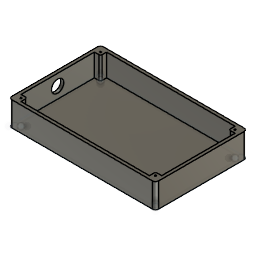
keyboard1_case (Autodesk Fusion 360 design; units mm, degrees)
part number: 2026-01-22-15-28-57-156
part number: 2026-01-22-16-58-12-345
part number: 2026-01-22-17-11-15-376
Autodesk Fusion 360 part; units mm, degrees
note: some values were not read from the file. Set by a fixed rule: which sketch regions a step uses.
sketch "bottom structure" plane through (0, 0, 0) normal (0, 0, 1) x (1, 0, 0)
  line L0 (5, 0) -> (235, 0)
  line L1 (240, 5) -> (240, 145)
  line L2 (235, 150) -> (5, 150)
  line L3 (0, 145) -> (0, 5)
  line L4 (10, 145) -> (230, 145)
  line L5 (235, 140) -> (235, 10)
  line L6 (230, 5) -> (10, 5)
  line L7 (5, 10) -> (5, 140)
  arc A0 (5, 150) -> (0, 145) centre (5, 145) ccw
  arc A1 (10, 145) -> (5, 140) centre (10, 140) ccw
  arc A2 (5, 10) -> (10, 5) centre (10, 10) ccw
  arc A3 (0, 5) -> (5, 0) centre (5, 5) ccw
  arc A4 (235, 140) -> (230, 145) centre (230, 140) ccw
  arc A5 (240, 145) -> (235, 150) centre (235, 145) ccw
  arc A6 (230, 5) -> (235, 10) centre (230, 10) ccw
  arc A7 (235, 0) -> (240, 5) centre (235, 5) ccw
  line L8 (15, 145) -> (15, 137.5)
  line L9 (12.5, 135) -> (5, 135)
  line L10 (225, 145) -> (225, 137.5)
  line L11 (227.5, 135) -> (235, 135)
  line L12 (5, 15) -> (12.5, 15)
  line L13 (15, 12.5) -> (15, 5)
  line L14 (225, 5) -> (225, 12.5)
  line L15 (227.5, 15) -> (235, 15)
  circle A8 centre (230, 10) radius 3
  circle A9 centre (230, 140) radius 3
  circle A10 centre (230, 140) radius 1.35
  circle A11 centre (10, 140) radius 1.35
  circle A12 centre (10, 140) radius 3
  circle A13 centre (230, 10) radius 1.35
  circle A14 centre (10, 10) radius 1.35
  circle A15 centre (10, 10) radius 3
  arc A16 (225, 137.5) -> (227.5, 135) centre (227.5, 137.5) ccw
  arc A17 (227.5, 15) -> (225, 12.5) centre (227.5, 12.5) ccw
  arc A18 (15, 12.5) -> (12.5, 15) centre (12.5, 12.5) ccw
  arc A19 (12.5, 135) -> (15, 137.5) centre (12.5, 137.5) ccw
  point P0 (240, 0)
  point P1 (0, 150)
  point P2 (15, 135)
  point P3 (225, 135)
  point P4 (15, 15)
  point P5 (225, 15)
  dimension "d1" = 150
  dimension "d2" = 240
  dimension "d4" = 5
  dimension "d5" = 5
  dimension "d6" = 5
  dimension "d7" = 5
  dimension "d8" = 5
  dimension "d9" = 5
  dimension "d10" = 5
  dimension "d11" = 5
  dimension "d12" = 5
  dimension "d13" = 5
  dimension "d14" = 5
  dimension "d15" = 5
  dimension "d16" = 10
  dimension "d17" = 10
  dimension "d18" = 10
  dimension "d19" = 10
  dimension "d20" = 10
  dimension "d21" = 10
  dimension "d22" = 10
  dimension "d23" = 10
  dimension "d24" = 5
  dimension "d25" = 6
  dimension "d27" = 5
  dimension "d31" = 6
  dimension "d34" = 2.7
  dimension "d35" = 6
  dimension "d36" = 2.7
  dimension "d38" = 2.7
  dimension "d39" = 6
  dimension "d40" = 2.7
  dimension "d41" = 2.5
  constraint horizontal L0
  constraint vertical L1
  constraint horizontal L2
  constraint vertical L3
  constraint horizontal L4
  constraint vertical L5
  constraint horizontal L6
  constraint vertical L7
  constraint coincident P1 L2
  constraint coincident P1 L3
  constraint tangent L2 A0
  constraint tangent L3 A0
  constraint tangent L4 A1
  constraint tangent L7 A1
  constraint tangent L6 A2
  constraint tangent L7 A2
  constraint coincident origin L0
  constraint coincident origin L3
  constraint tangent L0 A3
  constraint tangent L3 A3
  constraint tangent L4 A4
  constraint tangent L5 A4
  constraint tangent L1 A5
  constraint tangent L2 A5
  constraint tangent L5 A6
  constraint tangent L6 A6
  constraint coincident P0 L0
  constraint coincident P0 L1
  constraint tangent L0 A7
  constraint tangent L1 A7
  constraint coincident L4 L8.start
  constraint perpendicular L4 L8
  constraint coincident L7 L9.end
  constraint perpendicular L7 L9
  constraint coincident L4 L10.start
  constraint perpendicular L4 L10
  constraint coincident L5 L11.end
  constraint perpendicular L5 L11
  constraint coincident L7 L12.start
  constraint perpendicular L7 L12
  constraint coincident L6 L13.end
  constraint perpendicular L6 L13
  constraint coincident L6 L14.start
  constraint perpendicular L6 L14
  constraint coincident L5 L15.end
  constraint perpendicular L5 L15
  constraint coincident P3 L10
  constraint coincident P3 L11
  constraint tangent L10 A16
  constraint tangent L11 A16
  constraint coincident P5 L14
  constraint coincident P5 L15
  constraint tangent L14 A17
  constraint tangent L15 A17
  constraint equal A16 A17
  constraint coincident P4 L12
  constraint coincident P4 L13
  constraint tangent L12 A18
  constraint tangent L13 A18
  constraint equal A16 A18
  constraint coincident P2 L8
  constraint coincident P2 L9
  constraint tangent L8 A19
  constraint tangent L9 A19
  constraint equal A16 A19
  measures "d1" distance of origin P1
  measures "d2" distance of origin P0
  measures "d4" distance of L3 L7
  measures "d5" distance of L1 L5
  measures "d6" distance of L0 L6
  measures "d7" distance of L2 L4
  measures "d8" radius of A0
  measures "d9" radius of A1
  measures "d10" radius of A2
  measures "d11" radius of A3
  measures "d12" radius of A4
  measures "d13" radius of A5
  measures "d14" radius of A6
  measures "d15" radius of A7
  measures "d16" distance of L8.start P2
  measures "d17" distance of P2 L9.end
  measures "d18" distance of L10.start P3
  measures "d19" distance of P3 L11.end
  measures "d20" distance of L12.start P4
  measures "d21" distance of P4 L13.end
  measures "d22" distance of P5 L15.end
  measures "d23" distance of L14.start P5
  measures "d24" horizontal distance of L5.end A6.centre
  measures "d25" diameter of A8
  measures "d27" distance of L6.start A6.centre
  measures "d31" diameter of A9
  measures "d34" diameter of A10
  measures "d35" diameter of A12
  measures "d36" diameter of A11
  measures "d38" diameter of A13
  measures "d39" diameter of A15
  measures "d40" diameter of A14
  measures "d41" radius of A16
extrude "Extrude1" add sketch "bottom structure" along normal blind 40 contours L0 L1 L2 L3 A0 A3 A5 A7 | L4 L7 A1 L8 L9 A19 | L4 L5 A4 L10 L11 A16 | L6 L7 A2 L12 L13 A18 | L5 L6 A6 L14 L15 A17 | A8 | A9 | A12 | A15 makes body 1
sketch "bottom itself" plane through (0, 0, 0) normal (0, 0, 1) x (1, 0, 0)
  line L0 (5, 150) -> (235, 150)
  line L1 (240, 145) -> (240, 5)
  line L2 (235, 0) -> (5, 0)
  line L3 (0, 5) -> (0, 145)
  arc A0 (5, 150) -> (0, 145) centre (5, 145) ccw
  arc A1 (0, 5) -> (5, 0) centre (5, 5) ccw
  arc A2 (235, 0) -> (240, 5) centre (235, 5) ccw
  arc A3 (240, 145) -> (235, 150) centre (235, 145) ccw
  dimension "d44" = 5
  constraint horizontal L0
  constraint vertical L1
  constraint horizontal L2
  constraint vertical L3
  constraint tangent L0 A0
  constraint tangent L3 A0
  constraint tangent L2 A1
  constraint tangent L3 A1
  constraint equal A0 A1
  constraint tangent L1 A2
  constraint tangent L2 A2
  constraint equal A0 A2
  constraint tangent L0 A3
  constraint tangent L1 A3
  constraint equal A0 A3
  measures "d44" radius of A0
extrude "Extrude2" add sketch "bottom itself" along normal blind 5 bodies 1
extrude "Extrude3" cut 1 faces at (84.8596, 54.6296, 5) along direction (0, 0, -1) blind 1.5 on bodies 1 bodies 1
copy_body "Body->Comp1" bodies 1 removing the originals makes body 2 in component "top plate"
sketch "plate surface" plane through (0, 0, 40) normal (0, 0, 1) x (-1, 0, 0) in component "top plate"
  circle A0 centre (-10, -10) radius 1.35
  line L0 (-12.5, -15) -> (-5, -15)
  line L1 (-5, -15) -> (-5, -135)
  line L2 (-5, -135) -> (-12.5, -135)
  arc A1 (-12.5, -135) -> (-15, -137.5) centre (-12.5, -137.5) ccw
  line L3 (-15, -137.5) -> (-15, -145)
  line L4 (-15, -145) -> (-225, -145)
  line L5 (-225, -145) -> (-225, -137.5)
  arc A2 (-225, -137.5) -> (-227.5, -135) centre (-227.5, -137.5) ccw
  line L6 (-227.5, -135) -> (-235, -135)
  line L7 (-235, -135) -> (-235, -15)
  line L8 (-235, -15) -> (-227.5, -15)
  arc A3 (-227.5, -15) -> (-225, -12.5) centre (-227.5, -12.5) ccw
  line L9 (-225, -12.5) -> (-225, -5)
  line L10 (-225, -5) -> (-15, -5)
  line L11 (-15, -5) -> (-15, -12.5)
  arc A4 (-15, -12.5) -> (-12.5, -15) centre (-12.5, -12.5) ccw
  circle A5 centre (-10, -140) radius 1.35
  circle A6 centre (-230, -10) radius 1.35
  circle A7 centre (-230, -140) radius 1.35
  arc A8 (-235, 0) -> (-240, -5) centre (-235, -5) ccw
  line L12 (-240, -5) -> (-240, -145)
  arc A9 (-240, -145) -> (-235, -150) centre (-235, -145) ccw
  line L13 (-235, -150) -> (-5, -150)
  arc A10 (-5, -150) -> (0, -145) centre (-5, -145) ccw
  line L14 (0, -145) -> (0, -5)
  arc A11 (0, -5) -> (-5, 0) centre (-5, -5) ccw
  line L15 (-5, 0) -> (-235, 0)
  line L16 (-5, -150) -> (-235, -150)
  line L17 (-240, -145) -> (-240, -5)
  line L18 (-235, 0) -> (-5, 0)
  line L19 (0, -5) -> (0, -145)
  arc A12 (-5, -150) -> (0, -145) centre (-5, -145) ccw
  arc A13 (-240, -145) -> (-235, -150) centre (-235, -145) ccw
  arc A14 (-235, 0) -> (-240, -5) centre (-235, -5) ccw
  arc A15 (0, -5) -> (-5, 0) centre (-5, -5) ccw
  circle A16 centre (-230, -140) radius 1.65
  circle A17 centre (-230, -10) radius 1.65
  circle A18 centre (-10, -10) radius 1.65
  circle A19 centre (-10, -140) radius 1.65
  dimension "d49" = 5
  dimension "d50" = 5
  dimension "d51" = 5
  dimension "d52" = 5
  constraint horizontal L16
  constraint vertical L17
  constraint horizontal L18
  constraint vertical L19
  constraint tangent L16 A12
  constraint tangent L19 A12
  constraint tangent L16 A13
  constraint tangent L17 A13
  constraint tangent L17 A14
  constraint tangent L18 A14
  constraint tangent L18 A15
  constraint tangent L19 A15
  constraint concentric A7 A16
  constraint concentric A6 A17
  constraint concentric A0 A18
  constraint concentric A5 A19
  measures "d49" radius of A12
  measures "d50" radius of A13
  measures "d51" radius of A14
  measures "d52" radius of A15
extrude "Extrude1'" add sketch "plate surface" along normal blind 4 separate body contours L0 L1 L2 A1 L3 L4 L5 A2 L6 L7 L8 A3 L9 L10 L11 A4 | A8 L12 A9 L13 A10 L14 A11 L15 L16 L17 L18 L19 A12 A13 A14 A15 makes body 3 in component "plate"
sketch "hole" plane through (0, 0, 40) normal (0, 0, 1) x (-1, 0, 0) in component "top plate"
  circle A0 centre (-10, -10) radius 1.35
  line L0 (-12.5, -15) -> (-5, -15)
  line L1 (-5, -15) -> (-5, -135)
  line L2 (-5, -135) -> (-12.5, -135)
  arc A1 (-12.5, -135) -> (-15, -137.5) centre (-12.5, -137.5) ccw
  line L3 (-15, -137.5) -> (-15, -145)
  line L4 (-15, -145) -> (-225, -145)
  line L5 (-225, -145) -> (-225, -137.5)
  arc A2 (-225, -137.5) -> (-227.5, -135) centre (-227.5, -137.5) ccw
  line L6 (-227.5, -135) -> (-235, -135)
  line L7 (-235, -135) -> (-235, -15)
  line L8 (-235, -15) -> (-227.5, -15)
  arc A3 (-227.5, -15) -> (-225, -12.5) centre (-227.5, -12.5) ccw
  line L9 (-225, -12.5) -> (-225, -5)
  line L10 (-225, -5) -> (-15, -5)
  line L11 (-15, -5) -> (-15, -12.5)
  arc A4 (-15, -12.5) -> (-12.5, -15) centre (-12.5, -12.5) ccw
  circle A5 centre (-10, -140) radius 1.35
  circle A6 centre (-230, -10) radius 1.35
  circle A7 centre (-230, -140) radius 1.35
  arc A8 (-235, 0) -> (-240, -5) centre (-235, -5) ccw
  line L12 (-240, -5) -> (-240, -145)
  arc A9 (-240, -145) -> (-235, -150) centre (-235, -145) ccw
  line L13 (-235, -150) -> (-5, -150)
  arc A10 (-5, -150) -> (0, -145) centre (-5, -145) ccw
  line L14 (0, -145) -> (0, -5)
  arc A11 (0, -5) -> (-5, 0) centre (-5, -5) ccw
  line L15 (-5, 0) -> (-235, 0)
  line L16 (-61.7, -122.5) -> (-75.7, -122.5)
  line L17 (-75.7, -122.5) -> (-75.7, -108.5)
  line L18 (-75.7, -108.5) -> (-61.7, -108.5)
  line L19 (-61.7, -108.5) -> (-61.7, -122.5)
  line L20 (-29.5, -99) -> (-29.5, -85)
  line L21 (-29.5, -85) -> (-15.5, -85)
  line L22 (-15.5, -85) -> (-15.5, -99)
  line L23 (-15.5, -99) -> (-29.5, -99)
  line L24 (-99.5, -101.2) -> (-99.5, -87.2)
  line L25 (-99.5, -87.2) -> (-85.5, -87.2)
  line L26 (-85.5, -87.2) -> (-85.5, -101.2)
  line L27 (-85.5, -101.2) -> (-99.5, -101.2)
  line L28 (-49, -117) -> (-49, -103)
  line L29 (-49, -103) -> (-35, -103)
  line L30 (-35, -103) -> (-35, -117)
  line L31 (-35, -117) -> (-49, -117)
  line L32 (-109.5, -46) -> (-109.5, -32)
  line L33 (-109.5, -32) -> (-95.5, -32)
  line L34 (-95.5, -32) -> (-95.5, -46)
  line L35 (-95.5, -46) -> (-109.5, -46)
  line L36 (-144.5, -46) -> (-144.5, -32)
  line L37 (-144.5, -32) -> (-130.5, -32)
  line L38 (-130.5, -32) -> (-130.5, -46)
  line L39 (-130.5, -46) -> (-144.5, -46)
  line L40 (-154.5, -101.2) -> (-154.5, -87.2)
  line L41 (-154.5, -87.2) -> (-140.5, -87.2)
  line L42 (-140.5, -87.2) -> (-140.5, -101.2)
  line L43 (-140.5, -101.2) -> (-154.5, -101.2)
  line L44 (-178.3, -122.5) -> (-178.3, -108.5)
  line L45 (-178.3, -108.5) -> (-164.3, -108.5)
  line L46 (-164.3, -108.5) -> (-164.3, -122.5)
  line L47 (-164.3, -122.5) -> (-178.3, -122.5)
  line L48 (-205, -117) -> (-205, -103)
  line L49 (-205, -103) -> (-191, -103)
  line L50 (-191, -103) -> (-191, -117)
  line L51 (-191, -117) -> (-205, -117)
  line L52 (-224.5, -99) -> (-224.5, -85)
  line L53 (-224.5, -85) -> (-210.5, -85)
  line L54 (-210.5, -85) -> (-210.5, -99)
  line L55 (-210.5, -99) -> (-224.5, -99)
  dimension "d57" = 14
  dimension "d58" = 14
  dimension "d61" = 14
  dimension "d62" = 14
  dimension "d65" = 14
  dimension "d66" = 14
  dimension "d67" = 14
  dimension "d68" = 14
  dimension "d69" = 14
  dimension "d70" = 14
  dimension "d71" = 14
  dimension "d72" = 14
  dimension "d73" = 14
  dimension "d74" = 14
  dimension "d75" = 14
  dimension "d76" = 14
  dimension "d77" = 14
  dimension "d78" = 14
  dimension "d79" = 14
  dimension "d80" = 14
  dimension "d94" = 10.5
  dimension "d95" = 30
  dimension "d96" = 56.7
  dimension "d97" = 80.5
  dimension "d98" = 90.5
  dimension "d101" = 10.5
  dimension "d102" = 56.7
  dimension "d103" = 30
  dimension "d104" = 80.5
  dimension "d105" = 90.5
  dimension "d106" = 99
  dimension "d107" = 43.8
  dimension "d108" = 22.5
  dimension "d109" = 28
  dimension "d110" = 46
  dimension "d111" = 46
  dimension "d112" = 28
  dimension "d113" = 22.5
  dimension "d114" = 43.8
  dimension "d115" = 99
  constraint horizontal L16
  constraint vertical L17
  constraint horizontal L18
  constraint vertical L19
  constraint horizontal L23
  constraint vertical L20
  constraint horizontal L21
  constraint vertical L22
  constraint horizontal L27
  constraint vertical L24
  constraint horizontal L25
  constraint vertical L26
  constraint horizontal L31
  constraint vertical L28
  constraint horizontal L29
  constraint vertical L30
  constraint horizontal L35
  constraint vertical L32
  constraint horizontal L33
  constraint vertical L34
  constraint horizontal L39
  constraint vertical L36
  constraint horizontal L37
  constraint vertical L38
  constraint horizontal L43
  constraint vertical L40
  constraint horizontal L41
  constraint vertical L42
  constraint horizontal L47
  constraint vertical L44
  constraint horizontal L45
  constraint vertical L46
  constraint horizontal L51
  constraint vertical L48
  constraint horizontal L49
  constraint vertical L50
  constraint horizontal L55
  constraint vertical L52
  constraint horizontal L53
  constraint vertical L54
  measures "d57" distance of L16 L18
  measures "d58" distance of L17.end L18.end
  measures "d61" distance of L21 L23
  measures "d62" distance of L21.end L20.end
  measures "d65" distance of L25 L27
  measures "d66" distance of L25.end L24.end
  measures "d67" distance of L29 L31
  measures "d68" distance of L29.end L28.end
  measures "d69" distance of L33 L35
  measures "d70" distance of L33.end L32.end
  measures "d71" distance of L37 L39
  measures "d72" distance of L37.end L36.end
  measures "d73" distance of L41 L43
  measures "d74" distance of L41.end L40.end
  measures "d75" distance of L45 L47
  measures "d76" distance of L45.end L44.end
  measures "d77" distance of L49 L51
  measures "d78" distance of L49.end L48.end
  measures "d79" distance of L53 L55
  measures "d80" distance of L53.end L52.end
  measures "d94" distance of L7 L52
  measures "d95" distance of L7 L48
  measures "d96" distance of L7 L44
  measures "d97" distance of L7 L40
  measures "d98" distance of L7 L36
  measures "d101" distance of L1 L22
  measures "d102" distance of L1 L19
  measures "d103" distance of L1 L30
  measures "d104" distance of L1 L26
  measures "d105" distance of L1 L34
  measures "d106" distance of L4 L39
  measures "d107" distance of L4 L43
  measures "d108" distance of L4 L47
  measures "d109" distance of L4 L51
  measures "d110" distance of L4 L55
  measures "d111" distance of L4 L23
  measures "d112" distance of L4 L31
  measures "d113" distance of L4 L16
  measures "d114" distance of L4 L27
  measures "d115" distance of L4 L35
extrude "Extrude2'" cut sketch "hole" along normal blind 4 contours L16 L17 L18 L19 | L20 L21 L22 L23 | L24 L25 L26 L27 | L28 L29 L30 L31 | L32 L33 L34 L35 | L36 L37 L38 L39 | L40 L41 L42 L43 | L44 L45 L46 L47 | L48 L49 L50 L51 | L52 L53 L54 L55 bodies 3 in component "plate"
sketch "sink" plane through (0, 0, 40) normal (0, 0, 1) x (-1, 0, 0) in component "top plate"
  line L0 (-84.7, -86.4) -> (-100.3, -86.4)
  line L1 (-100.3, -86.4) -> (-100.3, -102)
  line L2 (-100.3, -102) -> (-84.7, -102)
  line L3 (-84.7, -102) -> (-84.7, -86.4)
  line L4 (-85.5, -87.2) -> (-99.5, -87.2)
  line L5 (-99.5, -87.2) -> (-99.5, -101.2)
  line L6 (-76.5, -107.7) -> (-76.5, -123.3)
  line L7 (-76.5, -123.3) -> (-60.9, -123.3)
  line L8 (-60.9, -107.7) -> (-76.5, -107.7)
  line L9 (-61.7, -108.5) -> (-75.7, -108.5)
  line L10 (-75.7, -108.5) -> (-75.7, -122.5)
  line L11 (-60.9, -123.3) -> (-60.9, -107.7)
  line L12 (-49.8, -102.2) -> (-49.8, -117.8)
  line L13 (-49.8, -117.8) -> (-34.2, -117.8)
  line L14 (-34.2, -102.2) -> (-49.8, -102.2)
  line L15 (-35, -103) -> (-49, -103)
  line L16 (-49, -103) -> (-49, -117)
  line L17 (-34.2, -117.8) -> (-34.2, -102.2)
  line L18 (-155.3, -86.4) -> (-155.3, -102)
  line L19 (-155.3, -102) -> (-139.7, -102)
  line L20 (-139.7, -86.4) -> (-155.3, -86.4)
  line L21 (-140.5, -87.2) -> (-154.5, -87.2)
  line L22 (-154.5, -87.2) -> (-154.5, -101.2)
  line L23 (-139.7, -102) -> (-139.7, -86.4)
  line L24 (-179.1, -107.7) -> (-179.1, -123.3)
  line L25 (-179.1, -123.3) -> (-163.5, -123.3)
  line L26 (-163.5, -107.7) -> (-179.1, -107.7)
  line L27 (-164.3, -108.5) -> (-178.3, -108.5)
  line L28 (-178.3, -108.5) -> (-178.3, -122.5)
  line L29 (-163.5, -123.3) -> (-163.5, -107.7)
  line L30 (-110.3, -31.2) -> (-110.3, -46.8)
  line L31 (-110.3, -46.8) -> (-94.7, -46.8)
  line L32 (-94.7, -31.2) -> (-110.3, -31.2)
  line L33 (-95.5, -32) -> (-109.5, -32)
  line L34 (-109.5, -32) -> (-109.5, -46)
  line L35 (-94.7, -46.8) -> (-94.7, -31.2)
  line L36 (-145.3, -31.2) -> (-145.3, -46.8)
  line L37 (-145.3, -46.8) -> (-129.7, -46.8)
  line L38 (-129.7, -31.2) -> (-145.3, -31.2)
  line L39 (-130.5, -32) -> (-144.5, -32)
  line L40 (-144.5, -32) -> (-144.5, -46)
  line L41 (-129.7, -46.8) -> (-129.7, -31.2)
  line L42 (-30.3, -84.2) -> (-30.3, -99.8)
  line L43 (-30.3, -99.8) -> (-14.7, -99.8)
  line L44 (-14.7, -84.2) -> (-30.3, -84.2)
  line L45 (-15.5, -85) -> (-29.5, -85)
  line L46 (-29.5, -85) -> (-29.5, -99)
  line L47 (-14.7, -99.8) -> (-14.7, -84.2)
  line L48 (-190.2, -117.8) -> (-190.2, -102.2)
  line L49 (-191, -103) -> (-205, -103)
  line L50 (-205.8, -117.8) -> (-190.2, -117.8)
  line L51 (-205.8, -102.2) -> (-205.8, -117.8)
  line L52 (-190.2, -102.2) -> (-205.8, -102.2)
  line L53 (-205, -103) -> (-205, -117)
  line L54 (-209.7, -99.8) -> (-209.7, -84.2)
  line L55 (-210.5, -85) -> (-224.5, -85)
  line L56 (-225.3, -99.8) -> (-209.7, -99.8)
  line L57 (-225.3, -84.2) -> (-225.3, -99.8)
  line L58 (-209.7, -84.2) -> (-225.3, -84.2)
  line L59 (-224.5, -85) -> (-224.5, -99)
  dimension "d118" = 15.6
  dimension "d119" = 15.6
  dimension "d120" = 0.8
  dimension "d121" = 0.8
  dimension "d122" = 15.6
  dimension "d123" = 15.6
  dimension "d124" = 0.8
  dimension "d125" = 0.8
  dimension "d126" = 15.6
  dimension "d127" = 15.6
  dimension "d128" = 0.8
  dimension "d129" = 0.8
  dimension "d130" = 15.6
  dimension "d131" = 15.6
  dimension "d132" = 0.8
  dimension "d133" = 0.8
  dimension "d134" = 15.6
  dimension "d135" = 15.6
  dimension "d136" = 0.8
  dimension "d137" = 0.8
  dimension "d138" = 15.6
  dimension "d139" = 15.6
  dimension "d140" = 0.8
  dimension "d141" = 0.8
  dimension "d142" = 15.6
  dimension "d143" = 15.6
  dimension "d144" = 0.8
  dimension "d145" = 0.8
  dimension "d146" = 15.6
  dimension "d147" = 15.6
  dimension "d148" = 0.8
  dimension "d149" = 0.8
  dimension "d150" = 15.6
  dimension "d151" = 15.6
  dimension "d152" = 0.8
  dimension "d153" = 0.8
  dimension "d154" = 15.6
  dimension "d155" = 15.6
  dimension "d156" = 0.8
  dimension "d157" = 0.8
  constraint horizontal L0
  constraint vertical L1
  constraint horizontal L2
  constraint vertical L3
  constraint horizontal L8
  constraint vertical L6
  constraint horizontal L7
  constraint vertical L11
  constraint horizontal L14
  constraint vertical L12
  constraint horizontal L13
  constraint vertical L17
  constraint horizontal L20
  constraint vertical L18
  constraint horizontal L19
  constraint vertical L23
  constraint horizontal L26
  constraint vertical L24
  constraint horizontal L25
  constraint vertical L29
  constraint horizontal L32
  constraint vertical L30
  constraint horizontal L31
  constraint vertical L35
  constraint horizontal L38
  constraint vertical L36
  constraint horizontal L37
  constraint vertical L41
  constraint horizontal L44
  constraint vertical L42
  constraint horizontal L43
  constraint vertical L47
  constraint horizontal L52
  constraint vertical L51
  constraint horizontal L50
  constraint vertical L48
  constraint horizontal L58
  constraint vertical L57
  constraint horizontal L56
  constraint vertical L54
  measures "d118" distance of L0.end L1.end
  measures "d119" distance of L0.start L0.end
  measures "d120" distance of L0 L4
  measures "d121" distance of L1 L5
  measures "d122" distance of L6.start L6.end
  measures "d123" distance of L8.start L6.start
  measures "d124" distance of L8 L9
  measures "d125" distance of L6 L10
  measures "d126" distance of L12.start L12.end
  measures "d127" distance of L14.start L12.start
  measures "d128" distance of L14 L15
  measures "d129" distance of L12 L16
  measures "d130" distance of L18.start L18.end
  measures "d131" distance of L20.start L18.start
  measures "d132" distance of L20 L21
  measures "d133" distance of L18 L22
  measures "d134" distance of L24.start L24.end
  measures "d135" distance of L26.start L24.start
  measures "d136" distance of L26 L27
  measures "d137" distance of L24 L28
  measures "d138" distance of L30.start L30.end
  measures "d139" distance of L32.start L30.start
  measures "d140" distance of L32 L33
  measures "d141" distance of L30 L34
  measures "d142" distance of L36.start L36.end
  measures "d143" distance of L38.start L36.start
  measures "d144" distance of L38 L39
  measures "d145" distance of L36 L40
  measures "d146" distance of L42.start L42.end
  measures "d147" distance of L44.start L42.start
  measures "d148" distance of L44 L45
  measures "d149" distance of L42 L46
  measures "d150" distance of L51.start L50.start
  measures "d151" distance of L48.end L51.start
  measures "d152" distance of L49 L52
  measures "d153" distance of L51 L53
  measures "d154" distance of L57.start L56.start
  measures "d155" distance of L54.end L57.start
  measures "d156" distance of L55 L58
  measures "d157" distance of L57 L59
extrude "Extrude3'" cut sketch "sink" along normal blind 2.5 bodies 3 in component "plate"
sketch "side hole" plane through (5, 0, 0) normal (1, 0, 0) x (0, 1, 0)
  line L0 (135, 3.5) -> (135, 40)
  line L1 (135, 40) -> (15, 40)
  line L2 (15, 40) -> (15, 3.5)
  line L3 (15, 3.5) -> (135, 3.5)
  circle A0 centre (75, 21.75) radius 10
  dimension "d160" = 20
  dimension "d161" = 60
  dimension "d162" = 18.25
  measures "d160" diameter of A0
  measures "d161" distance of L2 A0.centre
  measures "d162" distance of L3 A0.centre
extrude "Extrude1''" cut sketch "side hole" against normal blind 5 contours A0 bodies 2 in component "top plate"
component "top plate" placed x (1, 0, 0) y (0, 1, 0) z (0, 0, 1) at (0, 0, 0)
component "plate" placed x (1, 0, 0) y (0, 1, 0) z (0, 0, 1) at (0, 0, 0) in component "top plate"
